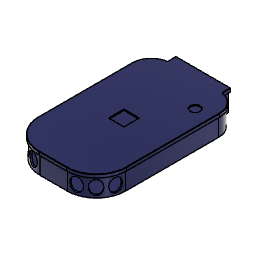
EsboçoFinal_v6 (Autodesk Fusion 360 design; units mm, degrees)
Autodesk Fusion 360 part; units mm, degrees
note: some values were not read from the file. Chosen so that the rebuilt part matches the saved one: which face or edge a step refers to.
sketch "Esboço1" plane through (0, 0, 0) normal (0, 0, 1) x (1, 0, 0)
  line L0 (-75, 95) -> (-75, -75)
  line L1 (-25, -125) -> (25, -125)
  line L2 (75, -75) -> (75, 95)
  line L3 (75, 125) -> (-75, -125) construction
  line L4 (-75, 125) -> (75, -125) construction
  arc A0 (-45, 125) -> (-75, 95) centre (-45, 95) ccw
  arc A1 (75, 95) -> (45, 125) centre (45, 95) ccw
  arc A2 (-75, -75) -> (-25, -125) centre (-25, -75) ccw
  arc A3 (25, -125) -> (75, -75) centre (25, -75) ccw
  line L5 (-45, 125) -> (-45, 140)
  line L6 (-45, 140) -> (45, 140)
  line L7 (45, 140) -> (45, 125)
  dimension "d3" = 150
  dimension "d4" = 250
  dimension "d5" = 30
  dimension "d6" = 30
  dimension "d7" = 50
  dimension "d8" = 50
  dimension "d9" = 90
  dimension "d10" = 15
  constraint parallel L0 L2
  constraint coincident L3 origin
  constraint coincident L4 origin
  constraint coincident L4.start L0
  constraint tangent L0 A0
  constraint coincident L3.start L2
  constraint tangent L2 A1
  constraint coincident L3.end L0
  constraint coincident L3.end L1
  constraint tangent L0 A2
  constraint tangent L1 A2
  constraint coincident L4.end L2
  constraint coincident L4.end L1
  constraint tangent L2 A3
  constraint tangent L1 A3
  constraint vertical L5
  constraint horizontal L6
  constraint vertical L7
  measures "d3" distance of L3.end L4.end
  measures "d4" distance of L4.start L3.end
  measures "d5" radius of A0
  measures "d6" radius of A1
  measures "d7" radius of A2
  measures "d8" radius of A3
  measures "d9" distance of A1.end A0.start
  measures "d10" distance of A1.end L6.end
extrude "Extrusão1" add sketch "Esboço1" along normal blind 30 makes body 1
shell "Casca1" thickness 3 outward yes removed faces 1 at (25, -18.333333, 30) on bodies 1
sketch "Esboço2" plane through (0, 143, 0) normal (0, 1, 0) x (-1, 0, 0)
  line L0 (-48, -3) -> (48, -3)
  line L1 (48, -3) -> (48, 30)
  line L2 (48, 30) -> (-48, 30)
  line L3 (-48, 30) -> (-48, -3)
  line L4 (-40, 25) -> (40, 25)
  line L5 (40, 25) -> (40, 5)
  line L6 (40, 5) -> (-40, 5)
  line L7 (-40, 5) -> (-40, 25)
  constraint horizontal L4
  constraint vertical L5
  constraint horizontal L6
  constraint vertical L7
extrude "Extrusão2" cut sketch "Esboço2" against normal blind 6 contours L4 L5 L6 L7 picked at (-13.333333, 18.333333) bodies 1
sketch "Esboço3" plane through (-78, 0, 0) normal (-1, 0, 0) x (0, -1, 0)
  line L0 (-95, -3) -> (75, -3)
  line L1 (75, -3) -> (75, 30)
  line L2 (75, 30) -> (-95, 30)
  line L3 (-95, 30) -> (-95, -3)
  line L4 (-28.690249, 24.6) -> (-79.690249, 24.6)
  line L5 (-79.690249, 24.6) -> (-79.690249, 2.4)
  line L6 (-79.690249, 2.4) -> (-28.690249, 2.4)
  line L7 (-28.690249, 2.4) -> (-28.690249, 24.6)
  line L8 (-28.690249, 24.6) -> (-79.690249, 2.4) construction
  line L9 (-79.690249, 24.6) -> (-28.690249, 2.4) construction
  point P0 (-54.190249, 13.5)
  dimension "d16" = 51
  dimension "d17" = 22.2
  constraint horizontal L4
  constraint perpendicular L4 L5
  constraint parallel L4 L6
  constraint parallel L5 L7
extrude "Extrusão3" cut sketch "Esboço3" against normal blind 6 contours L4 L5 L6 L7 picked at (-45.690249, 17.2) bodies 1
ref_plane "Plano de trabalho1" through (-75.127192, -92.21234, 14.331399) normal (-0.945796, -0.324761, 0) x (-0.324761, 0.945796, 0)
sketch "Esboço4" plane through (-75.127192, -92.21234, 14.331399) normal (-0.945796, -0.324761, 0) x (-0.324761, 0.945796, 0)
  ellipse E0 centre (0, 0) end of major axis (0, -12.5) minor radius 10.206437
  line L0 (0, 12.5) -> (0, -12.5)
  line L1 (-10.206437, 0) -> (10.206437, 0)
  dimension "d21" = 25
  constraint coincident E0 L0.start
  constraint coincident E0 L0.end
  constraint coincident E0.centre origin
  constraint vertical L0
  measures "d21" distance of E0
ref_plane "Plano de trabalho2" through (-63.713396, -111.197693, 20.395024) normal (-0.730441, -0.682975, 0) x (-0.682975, 0.730441, 0)
sketch "Esboço5" plane through (-63.713396, -111.197693, 20.395024) normal (-0.730441, -0.682975, 0) x (-0.682975, 0.730441, 0)
  ellipse E0 centre (-2.754765, 5.968658) end of major axis (-2.754765, 18.468658) minor radius 10
  line L0 (-2.754765, -6.531342) -> (-2.754765, 18.468658)
  line L1 (7.245235, 5.968658) -> (-12.754765, 5.968658)
  dimension "d23" = 25
  dimension "d24" = 20
  constraint vertical L0
  measures "d23" distance of E0
ref_plane "Plano de trabalho3" through (-39.926698, -125.854633, 10.618224) normal (-0.281636, -0.959521, 0) x (-0.959521, 0.281636, 0)
sketch "Esboço6" plane through (-39.926698, -125.854633, 10.618224) normal (-0.281636, -0.959521, 0) x (-0.959521, 0.281636, 0)
  ellipse E0 centre (0.306085, -3.826063) end of major axis (0.306085, 8.673937) minor radius 10
  line L0 (0.306085, -16.326063) -> (0.306085, 8.673937)
  line L1 (10.306085, -3.826063) -> (-9.693915, -3.826063)
  dimension "d26" = 25
  dimension "d27" = 20
  constraint vertical L0
  measures "d26" distance of E0
extrude "Extrusão4" cut sketch "Esboço6" against normal blind 6 bodies 1
extrude "Extrusão5" cut sketch "Esboço5" against normal blind 6 bodies 1
extrude "Extrusão6" cut sketch "Esboço4" against normal blind 6 bodies 1
ref_plane "Plano de trabalho5" through (76.486843, -87.57398, 11.382115) normal (0.97145, -0.237245, 0) x (-0.237245, -0.97145, 0)
sketch "Esboço7" plane through (76.486843, -87.57398, 11.382115) normal (0.97145, -0.237245, 0) x (-0.237245, -0.97145, 0)
ref_plane "Plano de trabalho6" through (58.370015, -116.175746, 13.5) normal (0.629623, -0.776901, 0) x (0.776901, 0.629623, 0)
sketch "Esboço8" plane through (58.370015, -116.175746, 13.5) normal (0.629623, -0.776901, 0) x (0.776901, 0.629623, 0)
  ellipse E0 centre (5, 0) end of major axis (5, 12.5) minor radius 10
  line L0 (5, -12.5) -> (5, 12.5)
  line L1 (15, 0) -> (-5, 0)
  dimension "d39" = 25
  dimension "d40" = 20
  constraint coincident E0 L0.start
  constraint coincident E0 L0.end
  constraint coincident E0 L1.start
  constraint coincident E0 L1.end
  constraint vertical L0
  measures "d39" distance of E0
ref_plane "Plano de trabalho7" through (36.575582, -126.720459, 13.662636) normal (0.218407, -0.975858, 0) x (-0.975858, -0.218407, 0)
sketch "Esboço9" plane through (36.575582, -126.720459, 13.662636) normal (0.218407, -0.975858, 0) x (-0.975858, -0.218407, 0)
  ellipse E0 centre (-2.631937, 0) end of major axis (-2.631937, -12.5) minor radius 10
  line L0 (-2.631937, 12.5) -> (-2.631937, -12.5)
  line L1 (-12.631937, 0) -> (7.368063, 0)
  dimension "d42" = 25
  dimension "d43" = 20
  constraint vertical L0
  measures "d42" distance of E0
ref_plane "Plano de trabalho8" through (76.531744, -87.388679, 0.189686) normal (0.972297, -0.233749, 0) x (-0.233749, -0.972297, 0)
sketch "Esboço10" plane through (76.531744, -87.388679, 0.189686) normal (0.972297, -0.233749, 0) x (-0.233749, -0.972297, 0)
  ellipse E0 centre (3, -13) end of major axis (3, -25.5) minor radius 10
  line L0 (3, -0.5) -> (3, -25.5)
  line L1 (-7, -13) -> (13, -13)
  dimension "d45" = 25
  dimension "d46" = 20
  constraint coincident E0 L0.start
  constraint coincident E0 L0.end
  constraint coincident E0 L1.start
  constraint coincident E0 L1.end
  constraint vertical L0
  measures "d45" distance of E0
extrude "Extrusão7" cut sketch "Esboço9" against normal blind 6 bodies 1
extrude "Extrusão8" cut sketch "Esboço8" against normal blind 6 bodies 1
extrude "Extrusão9" cut sketch "Esboço10" against normal blind 6 bodies 1
copy_body "Corpo -> Componente1" bodies 1 removing the originals makes body 2 in component "Component'"
sketch "Esboço4 (2)" plane through (0, 0, 0) normal (0, 0, 1) x (1, 0, 0) in component "Component''"
  arc A0 (-45, 125) -> (-75, 95) centre (-45, 95) ccw
  line L0 (-75, 95) -> (-75, -75)
  arc A1 (-75, -75) -> (-25, -125) centre (-25, -75) ccw
  line L1 (-25, -125) -> (25, -125)
  arc A2 (25, -125) -> (75, -75) centre (25, -75) ccw
  line L2 (75, -75) -> (75, 95)
  arc A3 (75, 95) -> (45, 125) centre (45, 95) ccw
  line L3 (45, 125) -> (45, 140)
  line L4 (45, 140) -> (-45, 140)
  line L5 (-45, 140) -> (-45, 125)
  line L6 (-45, 125) -> (-45, 140)
  line L7 (-45, 140) -> (45, 140)
  line L8 (45, 140) -> (45, 125)
  arc A4 (75, 95) -> (45, 125) centre (45, 95) ccw
  line L9 (75, 95) -> (75, -75)
  arc A5 (25, -125) -> (75, -75) centre (25, -75) ccw
  line L10 (25, -125) -> (-25, -125)
  arc A6 (-75, -75) -> (-25, -125) centre (-25, -75) ccw
  line L11 (-75, -75) -> (-75, 95)
  arc A7 (-45, 125) -> (-75, 95) centre (-45, 95) ccw
  arc A8 (-48, 127.863353) -> (-78, 95) centre (-45, 95) ccw
  line L12 (-78, 95) -> (-78, -75)
  arc A9 (-78, -75) -> (-25, -128) centre (-25, -75) ccw
  line L13 (-25, -128) -> (25, -128)
  arc A10 (25, -128) -> (78, -75) centre (25, -75) ccw
  line L14 (78, -75) -> (78, 95)
  arc A11 (78, 95) -> (48, 127.863353) centre (45, 95) ccw
  line L15 (48, 127.863353) -> (48, 143)
  line L16 (48, 143) -> (-48, 143)
  line L17 (-48, 143) -> (-48, 127.863353)
extrude "Extrusão1'" add sketch "Esboço4 (2)" along normal blind 34 separate body contours A0 L0 A1 L1 A2 L2 A3 L3 L4 L5 L6 L7 L8 A4 L9 A5 L10 A6 L11 A7 | A8 L12 A9 L13 A10 L14 A11 L15 L16 L17 picked at (25, -18.333333) picked at (-15, 142) makes body 3 in component "Component''"
extrude "Extrusão2'" cut 1 faces at (26, -18.333333, 34) along direction (0, 0, -1) blind 4 keep common part on bodies 3 bodies 3 in component "Component''"
sketch "Esboço5 (2)" plane through (0, 0, 34) normal (0, 0, 1) x (-1, 0, 0) in component "Component''"
  line L0 (48, -143) -> (48, -127.863353)
  arc A0 (48, -127.863353) -> (78, -95) centre (45, -95) ccw
  line L1 (78, -95) -> (78, 75)
  arc A1 (78, 75) -> (25, 128) centre (25, 75) ccw
  line L2 (25, 128) -> (-25, 128)
  arc A2 (-25, 128) -> (-78, 75) centre (-25, 75) ccw
  line L3 (-78, 75) -> (-78, -95)
  arc A3 (-78, -95) -> (-48, -127.863353) centre (-45, -95) ccw
  line L4 (-48, -127.863353) -> (-48, -143)
  line L5 (-48, -143) -> (48, -143)
shell "Casca1'" thickness 2 outward yes removed faces 1 at (26, -18.333333, 30) on bodies 3 in component "Component''"
fillet "Arredondamento1" radius 0.5 10 edges at (-50, 137.320508, 36) (-71.457513, 117.912878, 36) (-80, 10, 36) (-63.890873, -113.890873, 36) (0, -130, 36) (63.890873, -113.890873, 36) (80, 10, 36) (71.457513, 117.912878, 36) (50, 137.320508, 36) (0, 145, 36) on bodies 3 in component "Component''"
sketch "Esboço6 (2)" plane through (0, 0, 36) normal (0, 0, 1) x (-1, 0, 0) in component "Component''"
  arc A0 (49.5, -129.205263) -> (79.5, -95) centre (45, -95) ccw
  line L0 (79.5, -95) -> (79.5, 75)
  arc A1 (79.5, 75) -> (25, 129.5) centre (25, 75) ccw
  line L1 (25, 129.5) -> (-25, 129.5)
  arc A2 (-25, 129.5) -> (-79.5, 75) centre (-25, 75) ccw
  line L2 (-79.5, 75) -> (-79.5, -95)
  arc A3 (-79.5, -95) -> (-49.5, -129.205263) centre (-45, -95) ccw
  line L3 (-49.5, -129.205263) -> (-49.5, -144.5)
  line L4 (-49.5, -144.5) -> (49.5, -144.5)
  line L5 (49.5, -144.5) -> (49.5, -129.205263)
  circle A4 centre (-50, -80) radius 9
  line L6 (14, 14) -> (-14, 14)
  line L7 (-14, 14) -> (-14, -14)
  line L8 (-14, -14) -> (14, -14)
  line L9 (14, -14) -> (14, 14)
  line L10 (14, 14) -> (-14, -14) construction
  line L11 (-14, 14) -> (14, -14) construction
  dimension "d60" = 18
  dimension "d61" = 28
  dimension "d62" = 28
  constraint horizontal L6
  constraint perpendicular L6 L7
  constraint parallel L6 L8
  constraint parallel L7 L9
  constraint coincident L10 origin
  constraint coincident L11 origin
  measures "d60" diameter of A4
  measures "d61" distance of L7.end L8.end
  measures "d62" distance of L6.end L7.end
extrude "Extrusão3'" cut sketch "Esboço6 (2)" against normal blind 6 contours L6 L7 L8 L9 picked at (4.666667, 4.666667) bodies 3 in component "Component''"
extrude "Extrusão4'" cut sketch "Esboço6 (2)" against normal blind 6 contours A4 picked at (-47.608247, -75.964545) bodies 3 in component "Component''"
component "Component'" placed x (1, 0, 0) y (0, 1, 0) z (0, 0, 1) at (0, 0, 0)
component "Component''" placed x (1, 0, 0) y (0, 1, 0) z (0, 0, 1) at (0, 0, 0)
